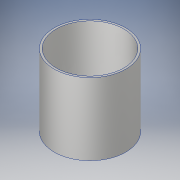
# Autodesk Inventor part: coso_pequeño
Saved by Autodesk Inventor 2019 (Build 230136000, 136)
## iProperties
Created: 2019-09-30
Part Number: coso_pequeño
Material: Aluminum 6061
Document SubType Name: Modeling
Designer: Domenico
Density: 2.7 g/cm^3
Appearance: Aluminum - Flat
diametro_externo: 28.575 mm
diametro_interno: 26.988 mm
Author: Domenico
Autodesk Inventor part; units mm, degrees
ref_plane "YZ Plane" through (0, 0, 0) normal (1, 0, 0) x (0, 1, 0)
ref_plane "XZ Plane" through (0, 0, 0) normal (0, 1, 0) x (-1, 0, 0)
ref_plane "XY Plane" through (0, 0, 0) normal (0, 0, 1) x (1, 0, 0)
sketch "Sketch1" plane through (0, 0, 0) normal (0, 1, 0) x (-1, 0, 0)
  circle A0 centre (0, 0) radius 14.2875
  circle A1 centre (0, 0) radius 13.4938
  dimension "diametro_externo" = 28.575
  dimension "diametro_interno" = 26.9875
  constraints: 2 centre point, 2 coincident
  measures "diametro_externo" diameter of A0
  measures "diametro_interno" diameter of A1
extrude "Extrusion1" add sketch "Sketch1" along normal blind 28.71
body "Solid1"
